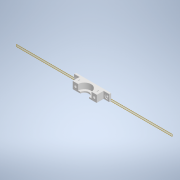
# Autodesk Inventor part: FrontPistonSupportButtom
Saved by Autodesk Inventor 2022.2 (Build 262287000, 287)
## iProperties
Created: 2022-02-15
Part Number: FrontPistonSupportButtom
Material: Generic
Document SubType Name: Modeling
Designer: siwat
Density: 1 g/cm^3
Appearance: Default
Author: siwat
Autodesk Inventor part; units mm, degrees
ref_plane "YZ Plane" through (0, 0, 0) normal (1, 0, 0) x (0, 1, 0)
ref_plane "XZ Plane" through (0, 0, 0) normal (0, 1, 0) x (-1, 0, 0)
ref_plane "XY Plane" through (0, 0, 0) normal (0, 0, 1) x (1, 0, 0)
ref_plane "Work Plane1" through (0, 0, 0) normal (0, 0, 1) x (1, 0, 0)
sketch "Sketch1" plane through (0, 0, 0) normal (0, 0, 1) x (1, 0, 0)
  line L0 (247.5, -5.2779) -> (147.5, -5.2779)
  line L1 (147.5, -5.2779) -> (147.5, 14.7221)
  line L2 (147.5, 14.7221) -> (247.5, 14.7221)
  line L3 (247.5, 14.7221) -> (247.5, -5.2779)
  line L4 (235, 40.7039) -> (235, 15.7039) projected
  line L5 (160, 15.7039) -> (160, 40.7039) projected
  line L6 (161, 181.7039) -> (234, 181.7039)
  arc A0 (235, 180.7039) -> (234, 181.7039) centre (234, 180.7039) ccw
  line L7 (235, 180.7039) -> (235, 155.7039)
  arc A1 (234, 154.7039) -> (235, 155.7039) centre (234, 155.7039) ccw
  line L8 (234, 154.7039) -> (219.9889, 154.7039)
  line L9 (219.9889, 154.7039) -> (219.9889, 41.7039)
  line L10 (219.9889, 41.7039) -> (234, 41.7039)
  arc A2 (235, 40.7039) -> (234, 41.7039) centre (234, 40.7039) ccw
  line L11 (235, 40.7039) -> (235, 15.7039)
  arc A3 (234, 14.7039) -> (235, 15.7039) centre (234, 15.7039) ccw
  line L12 (234, 14.7039) -> (229.5826, 14.7039)
  line L13 (229.5826, 14.7039) -> (229.5826, 21.7039)
  line L14 (229.5826, 21.7039) -> (220.4174, 21.7039)
  line L15 (220.4174, 21.7039) -> (220.4174, 14.7039)
  line L16 (220.4174, 14.7039) -> (174.5826, 14.7039)
  line L17 (174.5826, 14.7039) -> (174.5826, 21.7039)
  line L18 (174.5826, 21.7039) -> (165.4174, 21.7039)
  line L19 (165.4174, 21.7039) -> (165.4174, 14.7039)
  line L20 (165.4174, 14.7039) -> (161, 14.7039)
  arc A4 (160, 15.7039) -> (161, 14.7039) centre (161, 15.7039) ccw
  line L21 (160, 15.7039) -> (160, 40.7039)
  arc A5 (161, 41.7039) -> (160, 40.7039) centre (161, 40.7039) ccw
  line L22 (161, 41.7039) -> (175.0111, 41.7039)
  line L23 (175.0111, 41.7039) -> (175.0111, 154.7039)
  line L24 (175.0111, 154.7039) -> (161, 154.7039)
  arc A6 (160, 155.7039) -> (161, 154.7039) centre (161, 155.7039) ccw
  line L25 (160, 155.7039) -> (160, 180.7039)
  arc A7 (161, 181.7039) -> (160, 180.7039) centre (161, 180.7039) ccw
  line L26 (161, 181.7039) -> (234, 181.7039)
  arc A8 (235, 180.7039) -> (234, 181.7039) centre (234, 180.7039) ccw
  line L27 (235, 180.7039) -> (235, 155.7039)
  arc A9 (234, 154.7039) -> (235, 155.7039) centre (234, 155.7039) ccw
  line L28 (234, 154.7039) -> (219.9889, 154.7039)
  line L29 (219.9889, 154.7039) -> (219.9889, 41.7039)
  line L30 (219.9889, 41.7039) -> (234, 41.7039)
  arc A10 (235, 40.7039) -> (234, 41.7039) centre (234, 40.7039) ccw
  line L31 (235, 40.7039) -> (235, 15.7039)
  arc A11 (234, 14.7039) -> (235, 15.7039) centre (234, 15.7039) ccw
  line L32 (234, 14.7039) -> (229.5826, 14.7039)
  line L33 (229.5826, 14.7039) -> (229.5826, 21.7039)
  line L34 (229.5826, 21.7039) -> (220.4174, 21.7039)
  line L35 (220.4174, 21.7039) -> (220.4174, 14.7039)
  line L36 (220.4174, 14.7039) -> (174.5826, 14.7039)
  line L37 (174.5826, 14.7039) -> (174.5826, 21.7039)
  line L38 (174.5826, 21.7039) -> (165.4174, 21.7039)
  line L39 (165.4174, 21.7039) -> (165.4174, 14.7039)
  line L40 (165.4174, 14.7039) -> (161, 14.7039)
  arc A12 (160, 15.7039) -> (161, 14.7039) centre (161, 15.7039) ccw
  line L41 (160, 15.7039) -> (160, 40.7039)
  arc A13 (161, 41.7039) -> (160, 40.7039) centre (161, 40.7039) ccw
  line L42 (161, 41.7039) -> (175.0111, 41.7039)
  line L43 (175.0111, 41.7039) -> (175.0111, 154.7039)
  line L44 (175.0111, 154.7039) -> (161, 154.7039)
  arc A14 (160, 155.7039) -> (161, 154.7039) centre (161, 155.7039) ccw
  line L45 (160, 155.7039) -> (160, 180.7039)
  arc A15 (161, 181.7039) -> (160, 180.7039) centre (161, 180.7039) ccw
  line L46 (0, 0) -> (400, 0)
  line L47 (400, 0) -> (400, -5.0961)
  line L48 (0, -5.0961) -> (400, -5.0961)
  line L49 (0, -5.0961) -> (0, 0)
  line L50 (0, 14.5039) -> (400, 14.5039)
  line L51 (400, 14.5039) -> (400, 9.6864)
  line L52 (400, 9.6864) -> (0, 9.6864)
  line L53 (0, 9.6864) -> (0, 14.5039)
  circle A16 centre (240, 4.7221) radius 2.6
  circle A17 centre (155, 4.7221) radius 2.6
  point P0 (153.6248, 9.6864)
  point P1 (156.3752, 9.6864)
  point P2 (241.3752, 9.6864)
  point P3 (238.6248, 9.6864)
  dimension "d1" = 100
  dimension "d4" = -12.5
  dimension "d5" = 12.5
  dimension "d6" = 5.2
  dimension "d7" = 5.2
  dimension "d8" = 7.5
  dimension "d9" = 7.5
  dimension "d22" = 20
  dimension "d23" = 10
  dimension "d24" = 10
  constraints: 104 end point, 32 point on circle, 25 horizontal, 24 vertical, 18 centre point, 2 parallel, 1 perpendicular, 63 other
  measures "d1" distance of L0.start L0.end
  measures "d4" distance between parallel lines of L4 L3
  measures "d5" distance between parallel lines of L5 L1
  measures "d6" diameter of A16
  measures "d7" diameter of A17
  measures "d8" distance from line of L3 A16.centre
  measures "d9" distance from line of A17.centre L1
  measures "d22" distance of L2.end L0.start
  measures "d23" distance from line of A16.centre L0
  measures "d24" distance from line of A17.centre L0
extrude "Extrusion1" add sketch "Sketch1" along normal blind 5.3 contours L0 L1 L48 L3 | L48 L1 L46 L3 | L46 L1 L52 L3 | L52 L1 L50 L3 | L50 L1 L2 A4 L20 L19 L17 L16 L15 L13 L12 A3 L3 | A3 L12 L13 L2 | L2 L19 L20 A4 | L15 L16 L17 L2
sketch "Sketch2" plane through (147.5, -5.2779, 0) normal (0, -1, 0) x (1, 0, 0)
  circle A0 centre (50, 25.5) radius 19
  line L0 (69, 25.5) -> (84, 25.5)
  line L1 (31, 25.5) -> (16, 25.5)
  line L2 (16, 25.5) -> (16, 5.3)
  line L3 (0, 5.3) -> (100, 5.3) projected
  line L4 (84, 25.5) -> (84, 5.3)
  line L5 (84, 24.5) -> (68.9737, 24.5)
  line L6 (31.0263, 24.5) -> (16, 24.5)
  point P0 (-147.5, 0)
  dimension "d10" = 15
  dimension "d11" = 15
  dimension "d14" = 1
  constraints: 12 end point, 6 point on line, 4 point on circle, 3 horizontal, 2 line through centre, 2 perpendicular, 1 centre point, 2 other
  measures "d10" distance of L0.start L0.end
  measures "d11" distance of L1.start L1.end
  measures "d14" distance between parallel lines of L0 L5
extrude "Extrusion2" add sketch "Sketch2" against normal up to surface (20 mm away) contours L5 L4 L3 L2 L6 A0
sketch "Sketch3" plane through (216.4737, -5.2779, 24.5) normal (0, 0, 1) x (1, 0, 0)
  circle A0 centre (7.5263, 10) radius 3
  circle A1 centre (-45.4737, 10) radius 3
  line L0 (15.0263, 0) -> (15.0263, 20) projected
  line L1 (0, 0) -> (0, 20) projected
  line L2 (-52.9737, 0) -> (-52.9737, 20) projected
  line L3 (-37.9473, 0) -> (-52.9737, 0) projected
  line L4 (15.0263, 0) -> (0, 0) projected
  point P0 (-216.4737, 5.2779)
  point P1 (15.0263, 10)
  dimension "d15" = 6
  dimension "d16" = 6
  dimension "d17" = 7.5
  dimension "d19" = 7.5
  dimension "d25" = 10
  dimension "d26" = 10
  constraints: 2 centre point, 1 midpoint
  measures "d15" diameter of A0
  measures "d16" diameter of A1
  measures "d17" distance of point (15.026, 10) A0.centre
  measures "d19" distance from line of L2 A1.centre
  measures "d25" distance from line of L3 A1.centre
  measures "d26" distance from line of L4 A0.centre
extrude "Extrusion3" cut sketch "Sketch3" against normal blind 17
sketch "Sketch4" plane through (147.5, -5.2779, 0) normal (0, -1, 0) x (1, 0, 0)
  line L0 (84, 24.5) -> (68.9737, 24.5) projected
  line L1 (84, 24.5) -> (16, 24.5)
  line L2 (16, 24.5) -> (16, 5.3)
  line L3 (16, 5.3) -> (84, 5.3)
  line L4 (84, 5.3) -> (84, 24.5)
  arc A0 (31.0263, 24.5) -> (68.9737, 24.5) centre (50, 25.5) ccw projected
  circle A1 centre (50, 25.5) radius 12.5
  point P0 (-147.5, 0)
  point P1 (62.4599, 24.5)
  point P2 (37.5401, 24.5)
  dimension "d27" = 25
  constraints: 8 end point, 2 parallel, 1 centre point, 1 coincident, 1 horizontal, 1 perpendicular
  measures "d27" diameter of A1
extrude "Extrusion4" add sketch "Sketch4" against normal blind 4 contours L4 L3 L2 L1 A0 L0 | A0 L1 A1
sketch "Sketch5" plane through (147.5, -5.2779, 0) normal (0, -1, 0) x (1, 0, 0)
  line L0 (81, 16.5) -> (72, 16.5)
  line L1 (72, 16.5) -> (72, 11.5)
  line L2 (72, 11.5) -> (81, 11.5)
  line L3 (81, 11.5) -> (81, 16.5)
  line L4 (73.5, 24.5) -> (79.5, 24.5) projected
  line L5 (20.5, 24.5) -> (26.5, 24.5) projected
  line L6 (20.5, 7.5) -> (26.5, 7.5) projected
  line L7 (20.5, 24.5) -> (26.5, 24.5) projected
  line L8 (73.5, 7.5) -> (79.5, 7.5) projected
  line L9 (73.5, 24.5) -> (79.5, 24.5) projected
  line L10 (28, 16.5) -> (19, 16.5)
  line L11 (19, 16.5) -> (19, 11.5)
  line L12 (19, 11.5) -> (28, 11.5)
  line L13 (28, 11.5) -> (28, 16.5)
  point P0 (-147.5, 0)
  point P1 (76.5, 24.5)
  point P2 (76.5, 16.5)
  point P3 (23.5, 24.5)
  point P4 (23.5, 16.5)
  dimension "d30" = 9
  dimension "d31" = 5
  dimension "d32" = 6
  dimension "d33" = 1.5
  dimension "d34" = 8
  dimension "d35" = 9
  dimension "d36" = 5
  dimension "d37" = 6
  dimension "d38" = 1.5
  dimension "d39" = 8
  constraints: 16 end point, 4 midpoint, 4 parallel, 2 horizontal, 2 perpendicular
  measures "d30" distance of L2.end L1.end
  measures "d31" distance of L1.end L0.end
  measures "d32" distance of L8.start L8.end
  measures "d33" distance from line of L8.end L3
  measures "d34" distance of point (76.5, 24.5) point (76.5, 16.5)
  measures "d35" distance of L12.end L11.end
  measures "d36" distance of L11.end L10.end
  measures "d37" distance of L6.start L6.end
  measures "d38" distance from line of L6.end L13
  measures "d39" distance of point (23.5, 24.5) point (23.5, 16.5)
extrude "Extrusion5" cut sketch "Sketch5" against normal blind 15
sketch "Sketch6" plane through (147.5, 14.7221, 0) normal (0, 1, 0) x (1, 0, 0)
  line L0 (81, -11.5) -> (72, -11.5) projected
  line L1 (72, -11.5) -> (72, -16.5) projected
  line L2 (72, -16.5) -> (81, -16.5) projected
  line L3 (81, -16.5) -> (81, -11.5) projected
  line L4 (28, -11.5) -> (19, -11.5) projected
  line L5 (19, -11.5) -> (19, -16.5) projected
  line L6 (19, -16.5) -> (28, -16.5) projected
  line L7 (28, -16.5) -> (28, -11.5) projected
  line L8 (0, -5.3) -> (16, -5.3) projected
  line L9 (0, 0) -> (0, -5.3) projected
  line L10 (0, 0) -> (100, 0) projected
  line L11 (100, 0) -> (100, -5.3) projected
  line L12 (84, -5.3) -> (100, -5.3) projected
  line L13 (84, -5.3) -> (84, -24.5) projected
  line L14 (84, -24.5) -> (62.4599, -24.5) projected
  arc A0 (62.4599, -24.5) -> (37.5401, -24.5) centre (50, -25.5) ccw projected
  line L15 (37.5401, -24.5) -> (16, -24.5) projected
  line L16 (16, -24.5) -> (16, -5.3) projected
  line L17 (20.5, -11.5) -> (26.5, -11.5) projected
  line L18 (22, -11.5) -> (24, -11.5)
  line L19 (24, -11.5) -> (24, -16.5)
  line L20 (24, -16.5) -> (22, -16.5)
  line L21 (22, -16.5) -> (22, -11.5)
  line L22 (73.5, -11.5) -> (79.5, -11.5) projected
  line L23 (72, -16.5) -> (81, -16.5) projected
  line L24 (75, -11.5) -> (77, -11.5)
  line L25 (77, -11.5) -> (77, -16.5)
  line L26 (77, -16.5) -> (75, -16.5)
  line L27 (75, -16.5) -> (75, -11.5)
  point P0 (-147.5, 0)
  point P1 (22, -11.5)
  dimension "d42" = 2
  dimension "d43" = 9
  dimension "d44" = 3
  dimension "d45" = 2
  dimension "d46" = 3
  constraints: 16 end point, 4 parallel, 4 point on line, 2 horizontal, 2 perpendicular
  measures "d42" distance between parallel lines of L19 L21
  measures "d43" distance of L4.start L4.end
  measures "d44" distance between parallel lines of L5 L21
  measures "d45" distance of L25.end L26.end
  measures "d46" distance between parallel lines of L1 L27
extrude "Extrusion6" cut sketch "Sketch6" against normal through all contours L25 L2 L27 L0 | L19 L6 L21 L4
sketch "Sketch7" plane through (0, 0, 5.3) normal (0, 0, 1) x (1, 0, 0)
  circle A0 centre (240, 4.7221) radius 2.6 projected
  circle A1 centre (240, 4.7221) radius 5.75
  circle A2 centre (155, 4.7221) radius 2.6 projected
  circle A3 centre (155, 4.7221) radius 5.75
  point P0 (0, 0)
  dimension "d49" = 11.5
  dimension "d50" = 11.5
  constraints: 2 centre point, 2 coincident
  measures "d49" diameter of A1
  measures "d50" diameter of A3
extrude "Extrusion7" cut sketch "Sketch7" against normal blind 2
fillet "Fillet1" radius 1 12 edges at (239.5, -5.2779, 5.3) (231.5, -5.2779, 14.9) (163.5, -5.2779, 14.9) (147.5, 4.7221, 5.3) (155.5, 14.7221, 5.3) (155.5, -5.2779, 5.3) (247.5, 4.7221, 5.3) (239.5, 14.7221, 5.3) (247.5, 14.7221, 2.65) (247.5, -5.2779, 2.65) (147.5, -5.2779, 2.65) (147.5, 14.7221, 2.65)
equation "\"d30\" = d35"
equation "\"d31\" = d36"
equation "\"d33\" = -0.5 * d32 + 0.5 * d30"
equation "\"d34\" = d39"
equation "\"d38\" = -0.5 * d37 + 0.5 * d35"
equation "\"d49\" = d50"
body "Solid1"
